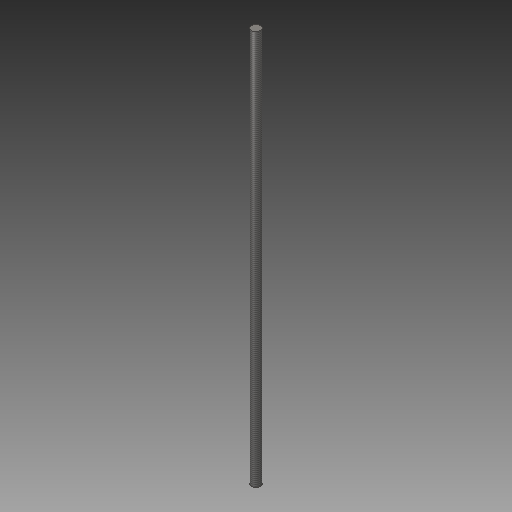
# Autodesk Inventor part: 350mmx8mm Lead Screw
Saved by Autodesk Inventor 2019 (Build 230136000, 136)
## iProperties
Created: 2018-10-12
Part Number: 350mmx8mm Lead Screw
Material: Stainless Steel
Document SubType Name: Modeling
Designer: Ax
Density: 8 g/cm^3
Appearance: Semi-Polished
Mass: 140.743 g
Surface Area: 88.9699 cm^2
Volume: 17.5929 cm^3
Author: Ax
Autodesk Inventor part; units mm, degrees
ref_plane "YZ Plane" through (0, 0, 0) normal (1, 0, 0) x (0, 1, 0)
ref_plane "XY Plane" through (0, 0, 0) normal (0, 0, 1) x (1, 0, 0)
sketch "Sketch1" plane through (0, 0, 0) normal (0, 1, 0) x (-1, 0, 0)
  circle A0 centre (0, 0) radius 4
  dimension "d0" = 8
  constraints: 1 centre point, 1 coincident
  measures "d0" diameter of A0
ref_plane "Work Plane4" through (0, 350, 0) normal (0, 1, 0) x (-1, 0, 0)
extrude "Extrusion2" add sketch "Sketch1" along normal up to surface (350 mm away)
thread "Thread2" size "TR8x1.5" class "7e" standard "ISO Metric Trapezoidal Threads" full length
body "Solid2"
